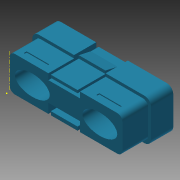
# Autodesk Inventor part: Connector Piece
Saved by Autodesk Inventor 2015 (Build 190159000, 159)
## iProperties
Created: 2014-10-27
Part Number: Connector Piece
Material: Generic
Document SubType Name: Modeling
Designer: cearhart275
Density: 1 g/cm^3
Appearance: Turquoise
Author: cearhart275
Autodesk Inventor part; units mm, degrees
ref_plane "YZ Plane" through (0, 0, 0) normal (1, 0, 0) x (0, 1, 0)
ref_plane "XZ Plane" through (0, 0, 0) normal (0, 1, 0) x (-1, 0, 0)
ref_plane "XY Plane" through (0, 0, 0) normal (0, 0, 1) x (1, 0, 0)
sketch "Sketch1" plane through (0, 0, 0) normal (0, 0, 1) x (1, 0, 0)
  line L0 (0, 20.0635) -> (57.9958, 20.0635)
  line L1 (57.9958, 20.0635) -> (57.9958, 0)
  line L2 (57.9958, 0) -> (0, 0)
  line L3 (0, 0) -> (0, 20.0635)
  dimension "d0" = 57.9958
  dimension "d1" = 20.0635
  constraints: 8 end point, 2 parallel, 1 coincident, 1 horizontal, 1 perpendicular
  measures "d0" distance of L0.start L0.end
  measures "d1" distance of L2.end L0.start
extrude "Extrusion1" add sketch "Sketch1" along normal blind 23.3426
sketch "Sketch2" plane through (0, 0, 23.3426) normal (0, 0, 1) x (1, 0, 0)
  line L0 (0, 20.0635) -> (57.9958, 20.0635)
  line L1 (57.9958, 20.0635) -> (57.9958, 0)
  line L2 (57.9958, 0) -> (0, 0)
  line L3 (0, 0) -> (0, 20.0635)
  line L4 (56.5556, 18.6233) -> (1.4402, 18.6233)
  line L5 (1.4402, 18.6233) -> (1.4402, 1.4402)
  line L6 (1.4402, 1.4402) -> (56.5556, 1.4402)
  line L7 (56.5556, 1.4402) -> (56.5556, 18.6233)
  point P0 (0, 0)
  dimension "d4" = 1.4402
  constraints: 16 end point, 4 parallel, 2 perpendicular, 1 horizontal, 3 other
  measures "d4" distance between parallel lines of L0 L4
extrude "Extrusion2" cut sketch "Sketch2" against normal blind 12.5197
sketch "Sketch3" plane through (1.4402, 18.6233, 23.3426) normal (0, 1, 0) x (1, 0, 0)
  line L0 (0, 0) -> (0, 12.5197) construction
  line L1 (4.3688, 0) -> (4.3688, 2.54) construction
  line L2 (0, 0) -> (55.1155, 0) construction
  line L3 (4.3688, 2.54) -> (15.3162, 2.54)
  line L4 (15.3162, 2.54) -> (15.3162, 3.9599)
  line L5 (15.3162, 3.9599) -> (4.3688, 3.9599)
  line L6 (4.3688, 3.9599) -> (4.3688, 2.54)
  line L7 (55.1155, 0) -> (55.1155, 12.5197) projected
  line L8 (50.7467, 2.54) -> (39.7993, 2.54)
  line L9 (39.7993, 2.54) -> (39.7993, 3.9599)
  line L10 (39.7993, 3.9599) -> (50.7467, 3.9599)
  line L11 (50.7467, 3.9599) -> (50.7467, 2.54)
  point P0 (-1.4402, 23.3426)
  dimension "d9" = 4.3688
  dimension "d10" = 2.54
  dimension "d11" = 10.9474
  dimension "d12" = 1.4199
  dimension "d15" = 2.54
  dimension "d16" = 4.3688
  dimension "d17" = 10.9474
  dimension "d18" = 1.4199
  constraints: 18 end point, 4 parallel, 2 horizontal, 2 perpendicular, 1 coincident, 1 vertical
  measures "d9" distance from line of L0 L1.end
  measures "d10" distance from line of L2 L1.end
  measures "d11" distance of L4.end L5.end
  measures "d12" distance of L3.end L4.end
  measures "d15" distance from line of L8.start L2
  measures "d16" distance from line of L7 L8.start
  measures "d17" distance of L9.end L10.end
  measures "d18" distance of L8.end L9.end
extrude "Extrusion3" cut sketch "Sketch3" against normal blind 0.4826 contours L6 L5 L4 L3
extrude "Extrusion4" cut sketch "Sketch3" against normal blind 0.4826 contours L8 L9 L10 L11
sketch "Sketch4" plane through (1.4402, 1.4402, 23.3426) normal (0, -1, 0) x (1, 0, 0)
  line L0 (50.7467, -2.54) -> (39.7993, -2.54)
  line L1 (39.7993, -2.54) -> (39.7993, -3.9599)
  line L2 (39.7993, -3.9599) -> (50.7467, -3.9599)
  line L3 (50.7467, -3.9599) -> (50.7467, -2.54)
  line L4 (4.3688, -2.54) -> (15.3162, -2.54)
  line L5 (15.3162, -2.54) -> (15.3162, -3.9599)
  line L6 (15.3162, -3.9599) -> (4.3688, -3.9599)
  line L7 (4.3688, -3.9599) -> (4.3688, -2.54)
  point P0 (-1.4402, -23.3426)
  constraints: 16 end point, 4 parallel, 2 horizontal, 2 perpendicular
extrude "Extrusion5" cut sketch "Sketch4" against normal blind 0.4826
sketch "Sketch5" plane through (0, 0, 0) normal (0, 0, -1) x (-1, 0, 0)
  line L0 (-49.149, 13.5356) -> (-8.509, 13.5356)
  line L1 (-8.509, 13.5356) -> (-8.509, 5.6362)
  line L2 (-8.509, 5.6362) -> (-49.149, 5.6362)
  line L3 (-49.149, 5.6362) -> (-49.149, 13.5356)
  line L4 (0, 0) -> (0, 20.0635) projected
  dimension "d23" = 40.64
  dimension "d24" = 8.509
  dimension "d25" = 7.8994
  constraints: 8 end point, 2 parallel, 1 horizontal, 1 perpendicular
  measures "d23" distance of L0.start L0.end
  measures "d24" distance between parallel lines of L4 L1
  measures "d25" distance of L2.end L0.start
extrude "Extrusion6" cut sketch "Sketch5" against normal blind 8.0112
sketch "Sketch6" plane through (0, 20.0635, 0) normal (0, 1, 0) x (1, 0, 0)
  line L0 (21.5646, 1.939) -> (20.3581, 1.939)
  line L1 (20.3581, 1.939) -> (20.3581, -30.94)
  line L2 (20.3581, -30.94) -> (21.5646, -30.94)
  line L3 (21.5646, -30.94) -> (21.5646, 1.939)
  line L4 (34.5821, 1.939) -> (35.7886, 1.939)
  line L5 (35.7886, 1.939) -> (35.7886, -30.94)
  line L6 (35.7886, -30.94) -> (34.5821, -30.94)
  line L7 (34.5821, -30.94) -> (34.5821, 1.939)
  line L8 (1.4402, -23.3426) -> (1.4402, -10.8229) projected
  point P0 (0, 0)
  dimension "d28" = 20.1244
  dimension "d29" = 1.2065
  dimension "d30" = 13.0175
  dimension "d31" = 1.2065
  constraints: 16 end point, 4 parallel, 2 horizontal, 2 perpendicular, 2 point on line
  measures "d28" distance between parallel lines of L3 L8
  measures "d29" distance of L1.end L2.end
  measures "d30" distance between parallel lines of L7 L3
  measures "d31" distance of L4.start L4.end
extrude "Extrusion7" cut sketch "Sketch6" against normal blind 4.3459
sketch "Sketch7" plane through (0, 0, 10.8229) normal (0, 0, 1) x (1, 0, 0)
  line L0 (21.5646, 20.0635) -> (34.5821, 20.0635)
  line L1 (34.5821, 20.0635) -> (34.5821, 18.6233)
  line L2 (34.5821, 18.6233) -> (21.5646, 18.6233)
  line L3 (21.5646, 18.6233) -> (21.5646, 20.0635)
  point P0 (0, 0)
  constraints: 8 end point, 2 parallel, 1 horizontal, 1 perpendicular
extrude "Extrusion8" cut sketch "Sketch7" against normal blind 1.1151
sketch "Sketch8" plane through (21.5646, 20.0635, 0) normal (0, 1, 0) x (1, 0, 0)
  line L0 (13.0175, -9.7079) -> (13.0175, 0) projected
  line L1 (0, 0) -> (13.0175, 0)
  line L2 (13.0175, 0) -> (13.0175, -3.8354)
  line L3 (13.0175, -3.8354) -> (0, -3.8354)
  line L4 (0, -3.8354) -> (0, 0)
  point P0 (-21.5646, 0)
  dimension "d36" = 3.8354
  constraints: 8 end point, 2 parallel, 1 horizontal, 1 perpendicular, 1 point on line
  measures "d36" distance of L1.end L2.end
extrude "Extrusion9" cut sketch "Sketch8" against normal blind 1.2979
sketch "Sketch10" plane through (0, 0, 23.3426) normal (0, 0, 1) x (1, 0, 0)
  ellipse E0 centre (12.5146, 9.6571) end of major axis (20.9893, 9.6571) minor radius 4.9479
  line L0 (0, 0) -> (0, 20.0635) projected
  line L1 (1.4402, 18.6233) -> (1.4402, 1.4402) projected
  line L2 (49.149, 13.5356) -> (8.509, 13.5356) projected
  line L3 (20.3581, 18.6233) -> (1.4402, 18.6233) projected
  ellipse E1 centre (45.4838, 9.6571) end of major axis (53.9585, 9.6571) minor radius 4.9479
  line L4 (8.509, 5.6362) -> (49.149, 5.6362) projected
  line L5 (35.7886, 20.0635) -> (57.9958, 20.0635) projected
  line L6 (56.5556, 18.6233) -> (35.7886, 18.6233) projected
  dimension "d41" = 8.4747
  dimension "d43" = 4.9479
  dimension "d51" = 4.9479
  dimension "d52" = 8.4747
  dimension "d44" = 11.0744
  dimension "d45" = 8.9662
  dimension "d49" = 32.9692
  dimension "d53" = 8.9662
  constraints: 1 horizontal, 4 other
  measures "d44" distance from line of L1 point (12.515, 9.657)
  measures "d45" distance from line of point (12.515, 9.657) L3
  measures "d49" distance of point (45.484, 9.657) point (12.515, 9.657)
  measures "d53" distance from line of L6 point (45.484, 9.657)
extrude "Extrusion10" cut sketch "Sketch10" against normal blind 11.9228 contours E0 | E1
sketch "Sketch11" plane through (0, 0, 23.3426) normal (0, 0, 1) x (1, 0, 0)
  line L0 (34.5821, 15.7175) -> (34.5821, 18.6233) projected
  line L1 (21.5646, 15.7175) -> (34.5821, 15.7175)
  line L2 (34.5821, 15.7175) -> (34.5821, 17.2745)
  line L3 (34.5821, 17.2745) -> (21.5646, 17.2745)
  line L4 (21.5646, 17.2745) -> (21.5646, 15.7175)
  line L5 (34.5821, 18.6233) -> (21.5646, 18.6233) projected
  point P0 (0, 0)
  dimension "d57" = 1.3487
  constraints: 8 end point, 2 parallel, 1 horizontal, 1 perpendicular, 1 point on line
  measures "d57" distance between parallel lines of L5 L3
extrude "Extrusion11" cut sketch "Sketch11" against normal blind 21.5265
sketch "Sketch12" plane through (34.5821, 18.6233, 9.7079) normal (1, 0, 0) x (0, 0, -1)
  line L0 (0, 1.4402) -> (5.8725, 0.1422)
  line L1 (5.8725, 0.1422) -> (5.8725, 1.4402)
  line L2 (9.7079, 1.4402) -> (-1.1151, 1.4402) projected
  line L3 (5.8725, 1.4402) -> (0, 1.4402)
  point P0 (9.7079, -18.6233)
  constraints: 6 end point, 2 perpendicular
extrude "Extrusion12" cut sketch "Sketch12" against normal up to next
sketch "Sketch13" plane through (0, 0, 23.3426) normal (0, 0, 1) x (1, 0, 0)
  line L0 (1.4402, 18.6233) -> (1.4402, 1.4402) construction
  point P0 (0, 0)
sketch "Sketch14" plane through (0, 0, 23.3426) normal (0, 0, 1) x (1, 0, 0)
  line L0 (35.7886, 6.096) -> (34.5821, 6.096)
  line L1 (34.5821, 6.096) -> (34.5821, -2.3095)
  line L2 (34.5821, -2.3095) -> (35.7886, -2.3095)
  line L3 (35.7886, -2.3095) -> (35.7886, 6.096)
  line L4 (21.5646, 6.096) -> (20.3581, 6.096)
  line L5 (20.3581, 6.096) -> (20.3581, -4.7581)
  line L6 (20.3581, -4.7581) -> (21.5646, -4.7581)
  line L7 (21.5646, -4.7581) -> (21.5646, 6.096)
  line L8 (1.4402, 1.4402) -> (56.5556, 1.4402) projected
  point P0 (0, 0)
  dimension "d62" = 4.6558
  dimension "d63" = 4.6558
  constraints: 16 end point, 4 parallel, 2 horizontal, 2 perpendicular
  measures "d62" distance between parallel lines of L8 L0
  measures "d63" distance between parallel lines of L8 L4
extrude "Extrusion13" cut sketch "Sketch14" against normal blind 2514.6
sketch "Sketch15" plane through (21.5646, 0, 0) normal (0, -1, 0) x (1, 0, 0)
  line L0 (13.0175, 0) -> (0.1116, 0)
  line L1 (13.0175, 10.8229) -> (0, 10.8229) projected
  line L2 (13.0175, 0) -> (0, 0)
  line L3 (0, 0) -> (0, 4.5466)
  line L4 (0, 4.5466) -> (13.0175, 4.5466)
  line L5 (13.0175, 4.5466) -> (13.0175, 0)
  line L6 (0, 10.8229) -> (0, 0) projected
  point P0 (-21.5646, 0)
  dimension "d67" = 4.5466
  constraints: 10 end point, 2 parallel, 2 perpendicular, 1 horizontal
  measures "d67" distance of L2.end L3.end
extrude "Extrusion14" cut sketch "Sketch15" against normal blind 0.8915
sketch "Sketch16" plane through (21.5646, 1.4402, 23.3426) normal (-1, 0, 0) x (0, 0, 1)
  line L0 (-12.5197, -1.4402) -> (-18.796, -0.5486)
  line L1 (-18.796, -0.5486) -> (-18.796, -1.4402)
  line L2 (-18.796, -1.4402) -> (-12.5197, -1.4402)
  line L3 (-12.5197, -1.4402) -> (-18.796, -1.4402) projected
  point P0 (-23.3426, -1.4402)
  constraints: 6 end point, 1 collinear
extrude "Extrusion15" cut sketch "Sketch16" against normal up to next
sketch "Sketch17" plane through (0, 0, 23.3426) normal (0, 0, 1) x (1, 0, 0)
  line L0 (21.5646, 6.096) -> (34.5821, 6.096)
  line L1 (34.5821, 6.096) -> (34.5821, 3.2004)
  line L2 (34.5821, 3.2004) -> (21.5646, 3.2004)
  line L3 (21.5646, 3.2004) -> (21.5646, 6.096)
  point P0 (0, 0)
  dimension "d72" = 2.8956
  constraints: 8 end point, 2 parallel, 1 horizontal, 1 perpendicular
  measures "d72" distance of L0.end L1.end
extrude "Extrusion16" cut sketch "Sketch17" against normal blind 21.5011
fillet "Fillet1" radius 2.54 4 edges at (56.5556, 18.6233, 17.0828) (1.4402, 18.6233, 17.0828) (1.4402, 1.4402, 17.0828) (56.5556, 1.4402, 17.0828)
fillet "Fillet2" radius 3.175 4 edges at (57.9958, 20.0635, 5.4115) (0, 20.0635, 5.4115) (57.9958, 0, 5.4115) (0, 0, 5.4115)
equation "\"d16\" = d9"
equation "\"d17\" = d11"
equation "\"d18\" = d12"
equation "\"d31\" = d29"
equation "\"d51\" = d43"
equation "\"d52\" = d41"
equation "\"d53\" = d45"
equation "\"d63\" = d62"
body "Solid1"
